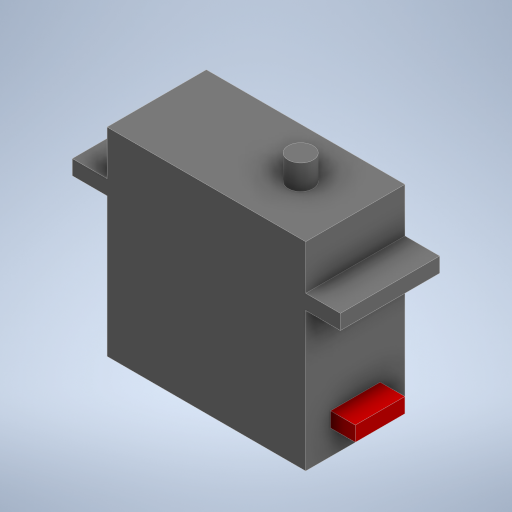
# Autodesk Inventor part: Servo_bigg_maketa
Saved by Autodesk Inventor 2023 (Build 270158000, 158)
## iProperties
Created: 2024-06-26
Part Number: Servo_bigg_maketa
Material: Generic
Document SubType Name: Modeling
Designer: Swoby
Density: 1 g/cm^3
Appearance: Default
Author: Swoby
Autodesk Inventor part; units mm, degrees
ref_plane "YZ Plane" through (0, 0, 0) normal (1, 0, 0) x (0, 1, 0)
ref_plane "XZ Plane" through (0, 0, 0) normal (0, 1, 0) x (-1, 0, 0)
sketch "Sketch1" plane through (0, 0, 0) normal (0, 0, 1) x (1, 0, 0)
  line L0 (-40, 0) -> (0, 0)
  line L1 (0, 0) -> (0, -7)
  line L2 (0, -7) -> (7, -7)
  line L3 (7, -7) -> (7, -10)
  line L4 (7, -10) -> (0, -10)
  line L5 (0, -10) -> (0, -30)
  line L6 (0, -38) -> (-40, -38)
  line L7 (-40, -38) -> (-40, -10)
  line L8 (-40, -10) -> (-47, -10)
  line L9 (-47, -10) -> (-47, -7)
  line L10 (-47, -7) -> (-40, -7)
  line L11 (-40, 0) -> (-40, -7)
  line L12 (0, -30) -> (5, -30)
  line L13 (5, -30) -> (5, -33)
  line L14 (5, -33) -> (0, -33)
  line L15 (0, -30) -> (0, -33) construction
  line L16 (0, -33) -> (0, -38)
  point P0 (7, -8.5)
  point P1 (-47, -8.5)
  point P2 (0, -24)
  dimension "d1" = 38
  dimension "d2" = 54
  dimension "d4" = 40
  dimension "d5" = 28
  dimension "d6" = 7
  dimension "d7" = 3
  dimension "d17" = 3
  dimension "d18" = 5
  dimension "d19" = 5
  constraints: 34 end point, 11 perpendicular, 8 point on line, 5 parallel, 2 horizontal, 2 midpoint, 1 coincident
  measures "d1" distance between parallel lines of L6 L0
  measures "d2" distance of point (7, -8.5) point (-47, -8.5)
  measures "d4" distance between parallel lines of L7 L5
  measures "d5" vertical distance of L6.end L8.end
  measures "d6" distance of L1.end L2.end
  measures "d7" distance of L2.end L3.end
  measures "d17" distance of L12.end L13.end
  measures "d18" distance of L5.end L12.end
  measures "d19" distance between parallel lines of L6 L14
extrude "Extrusion1" add sketch "Sketch1" along normal blind 20
sketch "Sketch2" plane through (-40, 0, 0) normal (0, 1, 0) x (1, 0, 0)
  circle A0 centre (29, -10) radius 2.5
  line L0 (-7, 0) -> (-7, -20) projected
  line L1 (40, 0) -> (40, -20) projected
  line L2 (40, -10) -> (0, -10) construction
  line L3 (0, 0) -> (0, -20) projected
  line L4 (40, 0) -> (0, 0) projected
  line L5 (0, 0) -> (0, -20) projected
  line L6 (40, -20) -> (0, -20) projected
  line L7 (40, 0) -> (40, -20) projected
  dimension "d11" = 5
  dimension "d12" = 36
  constraints: 2 end point, 2 midpoint, 1 centre point, 1 point on line
  measures "d11" diameter of A0
  measures "d12" distance from line of A0.centre L0
extrude "Extrusion2" add sketch "Sketch2" along normal blind 2 contours A0 | L1 L6 L3 L4
extrude "Extrusion3" add sketch "Sketch2" along normal blind 7 contours A0
sketch "Sketch3" plane through (0, -30, 0) normal (0, 1, 0) x (1, 0, 0)
  line L0 (5, 0) -> (0, 0) projected
  line L1 (0, 0) -> (0, -20) projected
  line L2 (5, -20) -> (0, -20) projected
  line L3 (5, 0) -> (5, -20) projected
  line L4 (0, 0) -> (0, -20) projected
  line L5 (5, 0) -> (5, -20) projected
  line L6 (0, -15) -> (5, -15)
  line L7 (5, -15) -> (5, -5)
  line L8 (5, -5) -> (0, -5)
  line L9 (0, -5) -> (0, -15)
  point P0 (0, -5)
  point P1 (5, -5)
  dimension "d20" = 5
  dimension "d21" = 5
  constraints: 8 end point, 2 parallel, 2 point on line, 1 horizontal, 1 perpendicular
  measures "d20" distance between parallel lines of L8 L0
  measures "d21" distance between parallel lines of L2 L6
extrude "Extrusion4" cut sketch "Sketch3" against normal through all contours L3 L8 L1 L0 | L3 L2 L1 L6
ref_plane "Work Plane1" through (0, 0, 10) normal (0, 0, 1) x (1, 0, 0)
body "Solid1"
